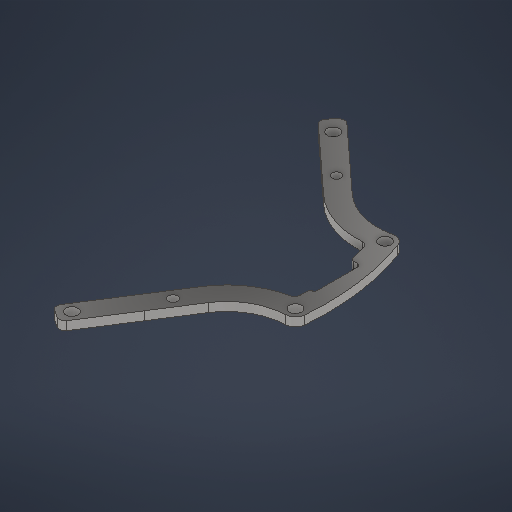
# Autodesk Inventor part: Schwungstrebe
Saved by Autodesk Inventor 2025.2 (Build 292293000, 293)
## iProperties
Created: 2024-05-17
Part Number: Schwungstrebe
Material: Generisch
Document SubType Name: Modeling
Designer: Fabian
Density: 1 g/cm^3
Appearance: Stahl - poliert
Author: Fabian
Autodesk Inventor part; units mm, degrees
ref_plane "YZ Plane" through (0, 0, 0) normal (1, 0, 0) x (0, 1, 0)
ref_plane "XZ Plane" through (0, 0, 0) normal (0, 1, 0) x (-1, 0, 0)
ref_plane "XY Plane" through (0, 0, 0) normal (0, 0, 1) x (1, 0, 0)
sketch "Skizze1" plane through (0, 0, 0) normal (0, 1, 0) x (-1, 0, 0)
  circle A0 centre (-82.6842, 7.2339) radius 2.1
  circle A1 centre (-82.6842, 7.2339) radius 2.1
  circle A2 centre (-77.9945, -28.3877) radius 2.1
  circle A3 centre (-77.9945, -28.3877) radius 2.1
  circle A4 centre (-49.9686, -39.6617) radius 1.6
  circle A5 centre (-49.9686, -39.6617) radius 1.6
  circle A6 centre (-58.5312, 25.3775) radius 1.6
  circle A7 centre (-58.5312, 25.3775) radius 1.6
  line L0 (-51.2809, 30.2441) -> (-59.8777, 16.7498)
  line L1 (-59.8777, 16.7498) -> (-65.7814, 20.5109)
  line L2 (-65.7814, 20.5109) -> (-57.1846, 34.0052)
  line L3 (-57.1846, 34.0052) -> (-51.2809, 30.2441)
  line L4 (-51.2809, 30.2441) -> (-65.7814, 20.5109) construction
  line L5 (-59.8777, 16.7498) -> (-57.1846, 34.0052) construction
  line L6 (13, 63) -> (-13, 63) construction
  line L7 (0, 63) -> (0, -88) construction
  arc A8 (-35.0888, -80.7018) -> (35.0888, -80.7018) centre (0, 0) ccw construction
  line L8 (0, 0) -> (-88, 0) construction
  arc A9 (-85.5688, 20.542) -> (-77.3365, -41.9889) centre (0, 0) ccw construction
  circle A10 centre (-82.6842, 7.2339) radius 3.5
  circle A11 centre (-77.9945, -28.3877) radius 3.5
  line L9 (-41.7058, -42.486) -> (-53.5023, -31.6766)
  line L10 (-53.5023, -31.6766) -> (-58.2314, -36.8375)
  line L11 (-58.2314, -36.8375) -> (-46.4349, -47.6469)
  line L12 (-46.4349, -47.6469) -> (-41.7058, -42.486)
  line L13 (-41.7058, -42.486) -> (-58.2314, -36.8375) construction
  line L14 (-53.5023, -31.6766) -> (-46.4349, -47.6469) construction
  arc A12 (-78.693, 11.2987) -> (-73.0957, -31.2612) centre (0, 0) ccw
  arc A13 (-86.1708, 7.539) -> (-81.2834, -29.5847) centre (0, 0) ccw
  arc A14 (-53.5023, -31.6766) -> (-77.9945, -24.8877) centre (-72.4082, -52.3088) ccw
  arc A15 (-58.2314, -36.8375) -> (-76.7973, -31.6766) centre (-72.5864, -52.5033) ccw
  arc A16 (-82.6842, 3.7339) -> (-59.8777, 16.7498) centre (-83.6316, 31.8827) ccw
  arc A17 (-82.6842, 10.7339) -> (-65.7814, 20.5109) centre (-83.642, 31.8893) ccw
  circle A18 centre (82.6842, 7.2339) radius 2.1
  circle A19 centre (82.6842, 7.2339) radius 2.1
  circle A20 centre (77.9945, -28.3877) radius 2.1
  circle A21 centre (77.9945, -28.3877) radius 2.1
  circle A22 centre (49.9686, -39.6617) radius 1.6
  circle A23 centre (49.9686, -39.6617) radius 1.6
  circle A24 centre (58.5312, 25.3775) radius 1.6
  circle A25 centre (58.5312, 25.3775) radius 1.6
  line L15 (51.2809, 30.2441) -> (59.8777, 16.7498)
  line L16 (59.8777, 16.7498) -> (65.7814, 20.5109)
  line L17 (65.7814, 20.5109) -> (57.1846, 34.0052)
  line L18 (57.1846, 34.0052) -> (51.2809, 30.2441)
  line L19 (51.2809, 30.2441) -> (65.7814, 20.5109) construction
  line L20 (59.8777, 16.7498) -> (57.1846, 34.0052) construction
  arc A26 (77.3365, -41.9889) -> (85.5688, 20.542) centre (0, 0) ccw construction
  circle A27 centre (82.6842, 7.2339) radius 3.5
  circle A28 centre (77.9945, -28.3877) radius 3.5
  line L21 (41.7058, -42.486) -> (53.5023, -31.6766)
  line L22 (53.5023, -31.6766) -> (58.2314, -36.8375)
  line L23 (58.2314, -36.8375) -> (46.4349, -47.6469)
  line L24 (46.4349, -47.6469) -> (41.7058, -42.486)
  line L25 (41.7058, -42.486) -> (58.2314, -36.8375) construction
  line L26 (53.5023, -31.6766) -> (46.4349, -47.6469) construction
  arc A29 (73.0957, -31.2612) -> (78.693, 11.2987) centre (0, 0) ccw
  arc A30 (81.2834, -29.5847) -> (86.1708, 7.539) centre (0, 0) ccw
  arc A31 (77.9945, -24.8877) -> (53.5023, -31.6766) centre (72.4082, -52.3088) ccw
  arc A32 (76.7973, -31.6766) -> (58.2314, -36.8375) centre (72.5864, -52.5033) ccw
  arc A33 (59.8777, 16.7498) -> (82.6842, 3.7339) centre (83.6316, 31.8827) ccw
  arc A34 (65.7814, 20.5109) -> (82.6842, 10.7339) centre (83.642, 31.8893) ccw
  arc A35 (54.3266, 20.6239) -> (52.9459, 20.93) centre (53.4832, 20.0866) ccw
  line L27 (52.9459, 20.93) -> (47.8855, 17.7062)
  arc A36 (47.8855, 17.7062) -> (47.5794, 16.3256) centre (48.4228, 16.8628) ccw
  line L28 (47.5794, 16.3256) -> (56.982, 1.5661)
  arc A37 (56.982, 1.5661) -> (58.3627, 1.26) centre (57.8254, 2.1034) ccw
  line L29 (58.3627, 1.26) -> (63.4231, 4.4838)
  arc A38 (63.4231, 4.4838) -> (63.7292, 5.8644) centre (62.8858, 5.3271) ccw
  line L30 (63.7292, 5.8644) -> (54.3266, 20.6239)
  arc A39 (45.7241, -33.9204) -> (47.137, -33.9821) centre (46.4614, -33.2448) ccw
  line L31 (47.137, -33.9821) -> (60.0395, -22.1594)
  arc A40 (60.0395, -22.1594) -> (60.1012, -20.7466) centre (59.3639, -21.4221) ccw
  line L32 (60.1012, -20.7466) -> (56.0477, -16.3229)
  arc A41 (56.0477, -16.3229) -> (54.6348, -16.2612) centre (55.3104, -16.9984) ccw
  line L33 (54.6348, -16.2612) -> (41.7323, -28.0839)
  arc A42 (41.7323, -28.0839) -> (41.6706, -29.4967) centre (42.4079, -28.8211) ccw
  line L34 (41.6706, -29.4967) -> (45.7241, -33.9204)
  circle A43 centre (30.623, 39.877) radius 2.1
  circle A44 centre (30.1839, -17.0814) radius 2.1
  circle A45 centre (46, -19.5) radius 1.375
  circle A46 centre (40, -19.5) radius 1.375
  circle A47 centre (40, 38.5) radius 1.375
  circle A48 centre (46, 38.5) radius 1.375
  arc A49 (-52.9459, 20.93) -> (-54.3266, 20.6239) centre (-53.4832, 20.0866) ccw
  line L35 (-54.3266, 20.6239) -> (-63.7292, 5.8644)
  arc A50 (-63.7292, 5.8644) -> (-63.4231, 4.4838) centre (-62.8858, 5.3271) ccw
  line L36 (-63.4231, 4.4838) -> (-58.3627, 1.26)
  arc A51 (-58.3627, 1.26) -> (-56.982, 1.5661) centre (-57.8254, 2.1034) ccw
  line L37 (-56.982, 1.5661) -> (-47.5794, 16.3256)
  arc A52 (-47.5794, 16.3256) -> (-47.8855, 17.7062) centre (-48.4228, 16.8628) ccw
  line L38 (-47.8855, 17.7062) -> (-52.9459, 20.93)
  arc A53 (-47.137, -33.9821) -> (-45.7241, -33.9204) centre (-46.4614, -33.2448) ccw
  line L39 (-45.7241, -33.9204) -> (-41.6706, -29.4967)
  arc A54 (-41.6706, -29.4967) -> (-41.7323, -28.0839) centre (-42.4079, -28.8211) ccw
  line L40 (-41.7323, -28.0839) -> (-54.6348, -16.2612)
  arc A55 (-54.6348, -16.2612) -> (-56.0477, -16.3229) centre (-55.3104, -16.9984) ccw
  line L41 (-56.0477, -16.3229) -> (-60.1012, -20.7466)
  arc A56 (-60.1012, -20.7466) -> (-60.0395, -22.1594) centre (-59.3639, -21.4221) ccw
  line L42 (-60.0395, -22.1594) -> (-47.137, -33.9821)
  arc A57 (-74.1912, 7.3101) -> (-74.5045, 6.2355) centre (-72.5045, 6.2355) ccw
  line L43 (-74.1912, 7.3101) -> (-66.8685, 18.8045)
  arc A58 (-66.8685, 18.8045) -> (-66.8312, 18.8624) centre (-71.8916, 22.0861) ccw
  line L44 (-66.8312, 18.8624) -> (-63.3633, 24.3059)
  arc A59 (-63.3633, 24.3059) -> (-63.3633, 24.306) centre (-65.0501, 25.3805) ccw
  line L45 (-63.3633, 24.306) -> (-61.5013, 27.2291)
  arc A60 (-61.5013, 27.2291) -> (-61.5073, 27.2194) centre (-58.5312, 25.3775) ccw
  line L46 (-61.5073, 27.2194) -> (-61.4583, 27.2963)
  arc A61 (-61.4583, 27.2963) -> (-61.4647, 27.2865) centre (-58.5312, 25.3775) ccw
  line L47 (-61.4647, 27.2865) -> (-59.6025, 30.2099)
  arc A62 (-59.6025, 30.2099) -> (-59.5849, 30.2371) centre (-61.2717, 31.3117) ccw
  line L48 (-59.5849, 30.2371) -> (-52.3622, 41.5746)
  arc A63 (-50.6754, 42.5) -> (-52.3622, 41.5746) centre (-50.6754, 40.5) ccw
  line L49 (-50.6754, 42.5) -> (-34.4476, 42.5)
  arc A64 (-34.4476, 42.5) -> (-33.1728, 42.959) centre (-34.4476, 44.5) ccw
  arc A65 (-28.0733, 42.959) -> (-33.1728, 42.959) centre (-30.623, 39.877) ccw
  arc A66 (-28.0733, 42.959) -> (-26.7984, 42.5) centre (-26.7984, 44.5) ccw
  line L50 (-26.7984, 42.5) -> (26.7984, 42.5)
  arc A67 (26.7984, 42.5) -> (28.0733, 42.959) centre (26.7984, 44.5) ccw
  arc A68 (33.1728, 42.959) -> (28.0733, 42.959) centre (30.623, 39.877) ccw
  arc A69 (33.1728, 42.959) -> (34.4476, 42.5) centre (34.4476, 44.5) ccw
  line L51 (34.4476, 42.5) -> (50.6754, 42.5)
  arc A70 (52.3622, 41.5746) -> (50.6754, 42.5) centre (50.6754, 40.5) ccw
  line L52 (52.3622, 41.5746) -> (59.5849, 30.2371)
  arc A71 (59.5849, 30.2371) -> (59.6025, 30.2099) centre (61.2717, 31.3117) ccw
  line L53 (59.6025, 30.2099) -> (61.4647, 27.2865)
  arc A72 (61.4647, 27.2865) -> (61.4583, 27.2963) centre (58.5312, 25.3775) ccw
  line L54 (61.4583, 27.2963) -> (61.5073, 27.2194)
  arc A73 (61.5073, 27.2194) -> (61.5013, 27.2291) centre (58.5312, 25.3775) ccw
  line L55 (61.5013, 27.2291) -> (63.3633, 24.306)
  arc A74 (63.3633, 24.306) -> (63.3633, 24.3059) centre (65.0501, 25.3805) ccw
  line L56 (63.3633, 24.3059) -> (66.8312, 18.8624)
  arc A75 (66.8312, 18.8624) -> (66.8685, 18.8045) centre (71.8916, 22.0861) ccw
  arc A76 (72.5045, -0.25) -> (74.5045, 1.75) centre (72.5045, 1.75) ccw
  line L57 (72.5045, -0.25) -> (63.2545, -0.25)
  arc A77 (63.2545, -0.25) -> (61.2545, -2.25) centre (63.2545, -2.25) ccw
  line L58 (61.2545, -2.25) -> (61.2545, -15.75)
  arc A78 (61.2545, -15.75) -> (63.2545, -17.75) centre (63.2545, -15.75) ccw
  line L59 (63.2545, -17.75) -> (72.5045, -17.75)
  arc A79 (74.5045, -19.75) -> (72.5045, -17.75) centre (72.5045, -19.75) ccw
  line L60 (74.5045, -19.75) -> (74.5045, -21.0459)
  arc A80 (73.8556, -22.5205) -> (74.5045, -21.0459) centre (72.5045, -21.0459) ccw
  arc A81 (51.2741, -42.5) -> (52.6253, -41.9746) centre (51.2741, -40.5) ccw
  line L61 (51.2741, -42.5) -> (-51.2741, -42.5)
  arc A82 (-52.6253, -41.9746) -> (-51.2741, -42.5) centre (-51.2741, -40.5) ccw
  line L62 (-52.6253, -41.9746) -> (-71.5045, -24.675)
  line L63 (-71.5045, -24.675) -> (-73.8556, -22.5205)
  arc A83 (-74.5045, -21.0459) -> (-73.8556, -22.5205) centre (-72.5045, -21.0459) ccw
  line L64 (-74.5045, -21.0459) -> (-74.5045, -19.75)
  arc A84 (-72.5045, -17.75) -> (-74.5045, -19.75) centre (-72.5045, -19.75) ccw
  line L65 (-72.5045, -17.75) -> (-63.2545, -17.75)
  arc A85 (-63.2545, -17.75) -> (-61.2545, -15.75) centre (-63.2545, -15.75) ccw
  line L66 (-61.2545, -15.75) -> (-61.2545, -2.25)
  arc A86 (-61.2545, -2.25) -> (-63.2545, -0.25) centre (-63.2545, -2.25) ccw
  line L67 (-63.2545, -0.25) -> (-72.5045, -0.25)
  arc A87 (-74.5045, 1.75) -> (-72.5045, -0.25) centre (-72.5045, 1.75) ccw
  line L68 (-74.5045, 1.75) -> (-74.5045, 6.2355)
  circle A88 centre (-46, 38.5) radius 1.375
  circle A89 centre (-40, 38.5) radius 1.375
  circle A90 centre (-40, -19.5) radius 1.375
  circle A91 centre (-46, -19.5) radius 1.375
  circle A92 centre (-30.1839, -17.0814) radius 2.1
  circle A93 centre (-30.623, 39.877) radius 2.1
  line L69 (44.0704, -45.0665) -> (38.9094, -49.7956) construction
  line L70 (47.6229, 42.5) -> (43.8618, 48.4037) construction
  line L71 (-47.6229, 42.5) -> (-43.8618, 48.4037) construction
  line L72 (-44.0704, -45.0665) -> (-38.9094, -49.7956) construction
  line L73 (31.3839, -51.9443) -> (41.7058, -42.486)
  line L74 (41.7058, -42.486) -> (46.4349, -47.6469)
  line L75 (46.4349, -47.6469) -> (36.1131, -57.1052)
  line L76 (36.1131, -57.1052) -> (31.3839, -51.9443)
  line L77 (31.3839, -51.9443) -> (46.4349, -47.6469) construction
  line L78 (41.7058, -42.486) -> (36.1131, -57.1052) construction
  line L79 (-31.3839, -51.9442) -> (-41.7058, -42.486)
  line L80 (-41.7058, -42.486) -> (-46.435, -47.647)
  line L81 (-46.435, -47.647) -> (-36.1131, -57.1052)
  line L82 (-36.1131, -57.1052) -> (-31.3839, -51.9442)
  line L83 (-31.3839, -51.9442) -> (-46.435, -47.647) construction
  line L84 (-41.7058, -42.486) -> (-36.1131, -57.1052) construction
  line L85 (38.9094, -49.7956) -> (33.7485, -54.5247)
  circle A94 centre (36.329, -52.1602) radius 2
  line L86 (33.7485, -54.5247) -> (32.2739, -55.8759)
  line L87 (32.2739, -55.8759) -> (34.6385, -58.4564)
  line L88 (34.6385, -58.4564) -> (36.1131, -57.1052)
  line L89 (32.2739, -55.8759) -> (29.9094, -53.2954)
  line L90 (29.9094, -53.2954) -> (31.3839, -51.9443)
  line L91 (-36.1131, -57.1052) -> (-31.3839, -51.9443)
  circle A95 centre (-36.329, -52.1602) radius 2
  line L92 (-33.7485, -54.5247) -> (-32.2739, -55.8759)
  line L93 (-32.2739, -55.8759) -> (-34.6385, -58.4564)
  line L94 (-34.6385, -58.4564) -> (-36.1131, -57.1052)
  line L95 (-32.2739, -55.8759) -> (-29.9094, -53.2954)
  line L96 (-29.9094, -53.2954) -> (-31.3839, -51.9443)
  line L97 (-40.9067, 53.0424) -> (-37.9548, 51.1618)
  line L98 (-37.9548, 51.1618) -> (-51.2809, 30.2441)
  line L99 (-40.9067, 53.0424) -> (-43.8585, 54.9229)
  line L100 (-43.8585, 54.9229) -> (-57.1846, 34.0052)
  circle A96 centre (-44.9364, 46.717) radius 2
  line L101 (-44.9364, 46.717) -> (-42.7872, 50.0905)
  line L102 (-42.7872, 50.0905) -> (-39.8354, 48.21)
  line L103 (-42.7872, 50.0905) -> (-45.7391, 51.9711)
  circle A97 centre (-44.9364, 46.717) radius 2.1
  circle A98 centre (-36.329, -52.1602) radius 2.1
  point P0 (0, 0)
  point P1 (-75.6274, -24.5102)
  point P2 (-79.3974, 4.0381)
  point P3 (-86.1708, 7.539)
  point P4 (-81.2834, -29.5847)
  point P5 (88, 0)
  point P6 (-41.6905, -42.5)
  point P7 (-41.7186, -42.5)
  dimension "d0" = 16
  dimension "d1" = 7
  dimension "d2" = 7
  dimension "d3" = 16
  dimension "d4" = 7
  dimension "d42" = 7
  dimension "d43" = 7
  dimension "d46" = 4
  dimension "d47" = 2
  dimension "d50" = 3.5
  dimension "d51" = 3.5
  dimension "d53" = 4
  dimension "d54" = 4
  dimension "d55" = 4.2
  dimension "d56" = 4.2
  constraints: 208 end point, 143 point on circle, 99 centre point, 40 symmetric about line, 22 coincident, 15 midpoint, 9 parallel, 9 perpendicular, 7 point on line, 5 tangent, 1 horizontal, 1 vertical, 18 other
  measures "d0" distance of L0.start L0.end
  measures "d1" diameter of A10
  measures "d2" diameter of A11
  measures "d3" distance of L9.start L9.end
  measures "d4" radial gap between concentric circles of A13 A12
  measures "d42" distance of L69.start L69.end
  measures "d43" distance of L70.start L70.end
  measures "d46" diameter of A94
  measures "d47" distance of L85.end L86.end
  measures "d50" distance of L97.start L97.end
  measures "d51" distance of L97.start L99.end
  measures "d53" diameter of A96
  measures "d54" distance of L101.start L101.end
  measures "d55" diameter of A97
  measures "d56" diameter of A98
extrude "Extrusion1" add sketch "Skizze1" along normal blind 3 contours L0 L1 L2 L3 | L3 L48 A63 L49 L98 A88 | A16 L68 A57 L43 A58 L44 L1 | A88 L98 | L44 A58 L43 A57 L68 A16 A12 A17 | L100 L103 L102 L98 L49 A63 | A12 A10 A17 | A16 A10 A12 | A12 A14 A11 A13 A10 A16 | A10 | A14 L63 L62 A15 A12 | A12 A11 A14 | A12 A15 A11 | A11 | A14 L10 L62 L63 | L9 L12 L61 A82 L11 L10 | L79 L61 L12 | A82 L61 L12 L11 | L61 L79 L82 L81 L12 | L96 L95 L92 L82 | L82 L92 L93 L94 picked at (-46.5547, 39.0575)
fillet "Rundung1" radius 2 6 edges at (79.3974, 1.5, 4.0381) (75.6274, 1.5, -24.5102) (29.9094, 1.5, -53.2954) (34.6385, 1.5, -58.4564) (45.7391, 1.5, 51.9711) (39.8354, 1.5, 48.21)
sketch "Skizze2" plane through (0, 3, 0) normal (0, 1, 0) x (1, 0, 0)
  line L0 (19.0016, 59.2215) -> (57.3401, 24.0908)
  arc A0 (57.3401, 24.0908) -> (69.3003, 22.9246) centre (64.096, 31.4636) ccw
  arc A1 (75.2406, 20.5635) -> (69.3003, 22.9246) centre (71.3821, 19.509) ccw
  arc A2 (77.999, -0.3892) -> (75.2406, 20.5635) centre (0, 0) ccw
  arc A3 (72.8723, -4.2072) -> (77.999, -0.3892) centre (73.9991, -0.3692) ccw
  arc A4 (72.8723, -4.2072) -> (61.6214, -8.4293) centre (70.0553, -13.8022) ccw
  line L1 (61.6214, -8.4293) -> (37.5911, -46.1492)
  arc A5 (34.2176, -48) -> (37.5911, -46.1492) centre (34.2176, -44) ccw
  line L2 (34.2176, -48) -> (29, -48)
  arc A6 (29, -48) -> (25.0078, -51.75) centre (29, -52) ccw
  arc A7 (21.0156, -55.5) -> (25.0078, -51.75) centre (21.0156, -51.5) ccw
  line L3 (21.0156, -55.5) -> (-21.0156, -55.5)
  circle A8 centre (36.75, -68) radius 1.8
  circle A9 centre (36.75, -61) radius 1.8
  circle A10 centre (36.75, -54) radius 1.8
  line L4 (30.1812, 62.5407) -> (59.6723, 35.5171)
  arc A11 (59.6723, 35.5171) -> (68.1495, 35.8873) centre (63.7258, 39.9408) ccw
  line L5 (68.1495, 35.8873) -> (74.1043, 42.3858)
  arc A12 (77.3365, 41.9889) -> (74.1043, 42.3858) centre (75.5788, 41.0346) ccw
  arc A13 (85.5688, -20.542) -> (77.3365, 41.9889) centre (0, 0) ccw
  arc A14 (82.5495, -21.7619) -> (85.5688, -20.542) centre (83.6241, -20.0751) ccw
  line L6 (82.5495, -21.7619) -> (75.1157, -17.026)
  arc A15 (75.1157, -17.026) -> (66.8315, -18.8626) centre (71.8919, -22.0864) ccw
  line L7 (66.8315, -18.8626) -> (45.3395, -52.5983)
  arc A16 (45.3395, -52.5983) -> (47.1761, -60.8824) centre (50.3999, -55.8221) ccw
  line L8 (47.1761, -60.8824) -> (54.6099, -65.6183)
  arc A17 (54.7803, -68.8703) -> (54.6099, -65.6183) centre (53.5353, -67.3051) ccw
  arc A18 (44.8368, -75.7209) -> (54.7803, -68.8703) centre (0, 0) ccw
  arc A19 (43.8178, -76) -> (44.8368, -75.7209) centre (43.8178, -74) ccw
  line L9 (43.8178, -76) -> (35.75, -76)
  arc A20 (33.75, -74) -> (35.75, -76) centre (35.75, -74) ccw
  line L10 (33.75, -74) -> (33.75, -64)
  arc A21 (33.75, -64) -> (30.0179, -63) centre (31.75, -64) ccw
  arc A22 (28.2859, -64) -> (30.0179, -63) centre (28.2859, -62) ccw
  line L11 (28.2859, -64) -> (14.7321, -64)
  circle A23 centre (49.9686, 39.6617) radius 1.8
  circle A24 centre (55.4982, 34.5948) radius 1.8
  circle A25 centre (58.5312, -25.3775) radius 1.8
  circle A26 centre (54.5014, -31.7029) radius 1.8
  circle A27 centre (62.5609, -19.052) radius 1.8
  line L12 (37.1695, -45.8805) -> (61.1997, -8.1606)
  arc A28 (73.0131, -3.7275) -> (61.1997, -8.1606) centre (70.0553, -13.8022) ccw
  arc A29 (73.0131, -3.7275) -> (77.499, -0.3867) centre (73.9991, -0.3692) ccw
  arc A30 (77.499, -0.3867) -> (74.7582, 20.4317) centre (0, 0) ccw
  arc A31 (74.7582, 20.4317) -> (69.5605, 22.4976) centre (71.3821, 19.509) ccw
  arc A32 (57.0023, 23.7222) -> (69.5605, 22.4976) centre (64.096, 31.4636) ccw
  line L13 (57.0023, 23.7222) -> (18.6638, 58.8529)
  line L14 (-21.0156, -55) -> (21.0156, -55)
  arc A33 (21.0156, -55) -> (24.5088, -51.7188) centre (21.0156, -51.5) ccw
  arc A34 (29, -47.5) -> (24.5088, -51.7188) centre (29, -52) ccw
  line L15 (29, -47.5) -> (34.2176, -47.5)
  arc A35 (34.2176, -47.5) -> (37.1695, -45.8805) centre (34.2176, -44) ccw
  line L16 (47.604, 37.0813) -> (31.5682, 51.7754)
  line L17 (31.5682, 51.7754) -> (63.6398, 22.3872)
  line L18 (63.6398, 22.3872) -> (50.128, 7.6416)
  line L19 (47.3023, 7.5183) -> (18.1798, 34.2041)
  line L20 (18.0564, 37.0298) -> (31.5682, 51.7754)
  line L21 (58.5312, -25.3775) -> (55.5793, -23.4969)
  line L22 (55.5793, -23.4969) -> (67.2656, -5.1532)
  line L23 (67.2656, -5.1532) -> (43.893, -41.8407)
  line L24 (43.893, -41.8407) -> (27.0252, -31.0947)
  line L25 (26.413, -28.3333) -> (47.6364, 4.9806)
  line L26 (50.3977, 5.5928) -> (67.2656, -5.1532)
  arc A36 (50.3977, 5.5928) -> (47.6364, 4.9806) centre (49.3231, 3.906) ccw
  arc A37 (47.3023, 7.5183) -> (50.128, 7.6416) centre (48.6535, 8.9928) ccw
  arc A38 (26.413, -28.3333) -> (27.0252, -31.0947) centre (28.0998, -29.4079) ccw
  line L27 (81.0045, 17) -> (62.0045, 17)
  line L28 (62.0045, 17) -> (62.0045, 1)
  line L29 (62.0045, 1) -> (81.0045, 1)
  line L30 (81.0045, 1) -> (81.0045, 17)
  line L31 (81.0045, 17) -> (62.0045, 1) construction
  line L32 (62.0045, 17) -> (81.0045, 1) construction
  arc A39 (-37.5911, -46.1492) -> (-34.2176, -48) centre (-34.2176, -44) ccw
  line L33 (-37.5911, -46.1492) -> (-61.6214, -8.4293)
  arc A40 (-61.6214, -8.4293) -> (-72.8723, -4.2072) centre (-70.0553, -13.8022) ccw
  arc A41 (-77.999, -0.3892) -> (-72.8723, -4.2072) centre (-73.9991, -0.3692) ccw
  arc A42 (-75.2406, 20.5635) -> (-77.999, -0.3892) centre (0, 0) ccw
  arc A43 (-69.3003, 22.9246) -> (-75.2406, 20.5635) centre (-71.3821, 19.509) ccw
  arc A44 (-69.3003, 22.9246) -> (-57.3401, 24.0908) centre (-64.096, 31.4636) ccw
  line L34 (-57.3401, 24.0908) -> (-19.0016, 59.2215)
  arc A45 (-19.0016, 59.2215) -> (-16.7974, 71.0346) centre (-25.7575, 66.5943) ccw
  arc A46 (-13.9276, 76.7465) -> (-16.7974, 71.0346) centre (-13.2134, 72.8108) ccw
  arc A47 (13.9276, 76.7465) -> (-13.9276, 76.7465) centre (0, 0) ccw
  arc A48 (16.7974, 71.0346) -> (13.9276, 76.7465) centre (13.2134, 72.8108) ccw
  arc A49 (16.7974, 71.0346) -> (19.0016, 59.2215) centre (25.7575, 66.5943) ccw
  line L35 (19.0016, 59.2215) -> (57.3401, 24.0908)
  arc A50 (57.3401, 24.0908) -> (69.3003, 22.9246) centre (64.096, 31.4636) ccw
  arc A51 (75.2406, 20.5635) -> (69.3003, 22.9246) centre (71.3821, 19.509) ccw
  arc A52 (77.999, -0.3892) -> (75.2406, 20.5635) centre (0, 0) ccw
  arc A53 (72.8723, -4.2072) -> (77.999, -0.3892) centre (73.9991, -0.3692) ccw
  arc A54 (72.8723, -4.2072) -> (61.6214, -8.4293) centre (70.0553, -13.8022) ccw
  line L36 (61.6214, -8.4293) -> (37.5911, -46.1492)
  arc A55 (34.2176, -48) -> (37.5911, -46.1492) centre (34.2176, -44) ccw
  line L37 (34.2176, -48) -> (29, -48)
  arc A56 (29, -48) -> (25.0078, -51.75) centre (29, -52) ccw
  arc A57 (21.0156, -55.5) -> (25.0078, -51.75) centre (21.0156, -51.5) ccw
  line L38 (21.0156, -55.5) -> (-21.0156, -55.5)
  arc A58 (-25.0078, -51.75) -> (-21.0156, -55.5) centre (-21.0156, -51.5) ccw
  arc A59 (-25.0078, -51.75) -> (-29, -48) centre (-29, -52) ccw
  line L39 (-29, -48) -> (-34.2176, -48)
  circle A60 centre (-24.9586, 79.1585) radius 2.8
  circle A61 centre (-76.682, 31.7627) radius 2.8
  circle A62 centre (-82.2899, -10.8337) radius 2.8
  circle A63 centre (-36.75, -68) radius 1.8
  circle A64 centre (-36.75, -61) radius 1.8
  circle A65 centre (-36.75, -54) radius 1.8
  circle A66 centre (-49.9686, 39.6617) radius 1.8
  circle A67 centre (-55.4982, 34.5948) radius 1.8
  circle A68 centre (-44.439, 44.7287) radius 1.8
  circle A69 centre (-62.5609, -19.052) radius 1.8
  circle A70 centre (-54.5014, -31.7029) radius 1.8
  circle A71 centre (-58.5312, -25.3775) radius 1.8
  circle A72 centre (36.75, -68) radius 1.8
  circle A73 centre (36.75, -61) radius 1.8
  circle A74 centre (36.75, -54) radius 1.8
  circle A75 centre (24.9586, 79.1585) radius 2.8
  arc A76 (29.8111, 71.018) -> (30.1812, 62.5407) centre (34.2347, 66.9644) ccw
  line L40 (30.1812, 62.5407) -> (59.6723, 35.5171)
  arc A77 (59.6723, 35.5171) -> (68.1495, 35.8873) centre (63.7258, 39.9408) ccw
  line L41 (68.1495, 35.8873) -> (74.1043, 42.3858)
  arc A78 (77.3365, 41.9889) -> (74.1043, 42.3858) centre (75.5788, 41.0346) ccw
  arc A79 (85.5688, -20.542) -> (77.3365, 41.9889) centre (0, 0) ccw
  arc A80 (82.5495, -21.7619) -> (85.5688, -20.542) centre (83.6241, -20.0751) ccw
  line L42 (82.5495, -21.7619) -> (75.1157, -17.026)
  arc A81 (75.1157, -17.026) -> (66.8315, -18.8626) centre (71.8919, -22.0864) ccw
  line L43 (66.8315, -18.8626) -> (45.3395, -52.5983)
  arc A82 (45.3395, -52.5983) -> (47.1761, -60.8824) centre (50.3999, -55.8221) ccw
  line L44 (47.1761, -60.8824) -> (54.6099, -65.6183)
  arc A83 (54.7803, -68.8703) -> (54.6099, -65.6183) centre (53.5353, -67.3051) ccw
  arc A84 (44.8368, -75.7209) -> (54.7803, -68.8703) centre (0, 0) ccw
  arc A85 (43.8178, -76) -> (44.8368, -75.7209) centre (43.8178, -74) ccw
  line L45 (43.8178, -76) -> (35.75, -76)
  arc A86 (33.75, -74) -> (35.75, -76) centre (35.75, -74) ccw
  line L46 (33.75, -74) -> (33.75, -64)
  arc A87 (33.75, -64) -> (30.0179, -63) centre (31.75, -64) ccw
  arc A88 (28.2859, -64) -> (30.0179, -63) centre (28.2859, -62) ccw
  line L47 (28.2859, -64) -> (14.7321, -64)
  arc A89 (13, -63) -> (14.7321, -64) centre (14.7321, -62) ccw
  line L48 (-14.7321, -64) -> (-28.2859, -64)
  arc A90 (-30.0179, -63) -> (-28.2859, -64) centre (-28.2859, -62) ccw
  arc A91 (-30.0179, -63) -> (-33.75, -64) centre (-31.75, -64) ccw
  line L49 (-33.75, -64) -> (-33.75, -74)
  arc A92 (-35.75, -76) -> (-33.75, -74) centre (-35.75, -74) ccw
  line L50 (-35.75, -76) -> (-43.8178, -76)
  arc A93 (-44.8368, -75.7209) -> (-43.8178, -76) centre (-43.8178, -74) ccw
  arc A94 (-54.7803, -68.8703) -> (-44.8368, -75.7209) centre (0, 0) ccw
  arc A95 (-54.6099, -65.6183) -> (-54.7803, -68.8703) centre (-53.5353, -67.3051) ccw
  line L51 (-54.6099, -65.6183) -> (-47.1761, -60.8824)
  arc A96 (-47.1761, -60.8824) -> (-45.3395, -52.5983) centre (-50.3999, -55.8221) ccw
  line L52 (-45.3395, -52.5983) -> (-66.8315, -18.8626)
  arc A97 (-66.8315, -18.8626) -> (-75.1157, -17.026) centre (-71.8919, -22.0864) ccw
  line L53 (-75.1157, -17.026) -> (-82.5495, -21.7619)
  arc A98 (-85.5688, -20.542) -> (-82.5495, -21.7619) centre (-83.6241, -20.0751) ccw
  arc A99 (-77.3365, 41.9889) -> (-85.5688, -20.542) centre (0, 0) ccw
  arc A100 (-74.1043, 42.3858) -> (-77.3365, 41.9889) centre (-75.5788, 41.0346) ccw
  line L54 (-74.1043, 42.3858) -> (-68.1495, 35.8873)
  arc A101 (-68.1495, 35.8873) -> (-59.6723, 35.5171) centre (-63.7258, 39.9408) ccw
  line L55 (-59.6723, 35.5171) -> (-30.1812, 62.5407)
  arc A102 (-30.1812, 62.5407) -> (-29.8111, 71.018) centre (-34.2347, 66.9644) ccw
  line L56 (-29.8111, 71.018) -> (-35.7659, 77.5165)
  arc A103 (-35.0888, 80.7018) -> (-35.7659, 77.5165) centre (-34.2913, 78.8676) ccw
  arc A104 (35.0888, 80.7018) -> (-35.0888, 80.7018) centre (0, 0) ccw
  arc A105 (35.7659, 77.5165) -> (35.0888, 80.7018) centre (34.2913, 78.8676) ccw
  line L57 (35.7659, 77.5165) -> (29.8111, 71.018)
  circle A106 centre (49.9686, 39.6617) radius 1.8
  circle A107 centre (55.4982, 34.5948) radius 1.8
  circle A108 centre (58.5312, -25.3775) radius 1.8
  circle A109 centre (54.5014, -31.7029) radius 1.8
  circle A110 centre (44.439, 44.7287) radius 1.8
  circle A111 centre (62.5609, -19.052) radius 1.8
  line L58 (37.1695, -45.8805) -> (61.1997, -8.1606)
  arc A112 (73.0131, -3.7275) -> (61.1997, -8.1606) centre (70.0553, -13.8022) ccw
  arc A113 (73.0131, -3.7275) -> (77.499, -0.3867) centre (73.9991, -0.3692) ccw
  arc A114 (77.499, -0.3867) -> (74.7582, 20.4317) centre (0, 0) ccw
  arc A115 (74.7582, 20.4317) -> (69.5605, 22.4976) centre (71.3821, 19.509) ccw
  arc A116 (57.0023, 23.7222) -> (69.5605, 22.4976) centre (64.096, 31.4636) ccw
  line L59 (57.0023, 23.7222) -> (18.6638, 58.8529)
  arc A117 (16.3494, 71.2566) -> (18.6638, 58.8529) centre (25.7575, 66.5943) ccw
  arc A118 (16.3494, 71.2566) -> (13.8384, 76.2545) centre (13.2134, 72.8108) ccw
  arc A119 (13.8384, 76.2545) -> (-13.8384, 76.2545) centre (0, 0) ccw
  arc A120 (-13.8384, 76.2545) -> (-16.3494, 71.2566) centre (-13.2134, 72.8108) ccw
  arc A121 (-18.6638, 58.8529) -> (-16.3494, 71.2566) centre (-25.7575, 66.5943) ccw
  line L60 (-18.6638, 58.8529) -> (-57.0023, 23.7222)
  arc A122 (-69.5605, 22.4976) -> (-57.0023, 23.7222) centre (-64.096, 31.4636) ccw
  arc A123 (-69.5605, 22.4976) -> (-74.7582, 20.4317) centre (-71.3821, 19.509) ccw
  arc A124 (-74.7582, 20.4317) -> (-77.499, -0.3867) centre (0, 0) ccw
  arc A125 (-77.499, -0.3867) -> (-73.0131, -3.7275) centre (-73.9991, -0.3692) ccw
  arc A126 (-61.1997, -8.1606) -> (-73.0131, -3.7275) centre (-70.0553, -13.8022) ccw
  line L61 (-61.1997, -8.1606) -> (-37.1695, -45.8805)
  arc A127 (-37.1695, -45.8805) -> (-34.2176, -47.5) centre (-34.2176, -44) ccw
  line L62 (-34.2176, -47.5) -> (-29, -47.5)
  arc A128 (-24.5088, -51.7188) -> (-29, -47.5) centre (-29, -52) ccw
  arc A129 (-24.5088, -51.7188) -> (-21.0156, -55) centre (-21.0156, -51.5) ccw
  line L63 (-21.0156, -55) -> (21.0156, -55)
  arc A130 (21.0156, -55) -> (24.5088, -51.7188) centre (21.0156, -51.5) ccw
  arc A131 (29, -47.5) -> (24.5088, -51.7188) centre (29, -52) ccw
  line L64 (29, -47.5) -> (34.2176, -47.5)
  arc A132 (34.2176, -47.5) -> (37.1695, -45.8805) centre (34.2176, -44) ccw
  circle A133 centre (16, 9) radius 2.1
  line L65 (-19, -53) -> (-19, 12)
  circle A134 centre (4, 47) radius 1.621
  circle A135 centre (-4, 47) radius 1.621
  arc A136 (7, 49.9161) -> (10.3333, 45.972) centre (11, 49.9161) ccw
  arc A137 (12, 44) -> (10.3333, 45.972) centre (10, 44) ccw
  line L66 (12, 44) -> (12, -5)
  line L67 (12, -5) -> (10, -5)
  arc A138 (8, -3) -> (10, -5) centre (10, -3) ccw
  line L68 (8, -3) -> (8, 1)
  arc A139 (8, 1) -> (6, 3) centre (6, 1) ccw
  line L69 (6, 3) -> (-6, 3)
  arc A140 (-6, 3) -> (-8, 1) centre (-6, 1) ccw
  line L70 (-8, 1) -> (-8, -3)
  arc A141 (-10, -5) -> (-8, -3) centre (-10, -3) ccw
  line L71 (-10, -5) -> (-12, -5)
  line L72 (-12, -5) -> (-12, 44)
  arc A142 (-10.3333, 45.972) -> (-12, 44) centre (-10, 44) ccw
  arc A143 (-10.3333, 45.972) -> (-7, 49.9161) centre (-11, 49.9161) ccw
  line L73 (-7, 49.9161) -> (-7, 54)
  arc A144 (-5, 56) -> (-7, 54) centre (-5, 54) ccw
  line L74 (-5, 56) -> (5, 56)
  arc A145 (7, 54) -> (5, 56) centre (5, 54) ccw
  line L75 (7, 54) -> (7, 49.9161)
  line L76 (-13, -63) -> (13, -63) construction
  line L77 (0, -63) -> (0, 88) construction
  arc A146 (35.0888, 80.7018) -> (-35.0888, 80.7018) centre (0, 0) ccw construction
  line L78 (0, 0) -> (88, 0) construction
  arc A147 (85.5688, -20.542) -> (77.3365, 41.9889) centre (0, 0) ccw construction
  circle A148 centre (0, 0) radius 75 construction
  line L79 (0, 0) -> (70.4769, 25.6515) construction
  line L80 (0, 0) -> (74.7146, -6.5367) construction
  circle A149 centre (0, 0) radius 78
  circle A150 centre (70.4769, 25.6515) radius 3
  circle A151 centre (74.7146, -6.5367) radius 3
  circle A152 centre (0, 0) radius 72
  arc A153 (29, -48) -> (25.0078, -51.75) centre (29, -52) ccw construction
  circle A154 centre (29, -52) radius 3.5
  line L81 (34.2176, -48) -> (29, -48) construction
  line L82 (29, -55.5) -> (21.0156, -55.5)
  circle A155 centre (29, -52) radius 4
  line L83 (32.5, -48) -> (29, -48)
  arc A156 (21.0156, -55.5) -> (25.0078, -51.75) centre (21.0156, -51.5) ccw
  arc A157 (21.0156, -55.5) -> (25.0078, -51.75) centre (21.0156, -51.5) ccw
  line L84 (32.5, -52) -> (32.5, -48)
  circle A158 centre (74.7146, -6.5367) radius 1.6
  circle A159 centre (70.4769, 25.6515) radius 1.6
  circle A160 centre (29, -52) radius 1.6
  line L85 (0, -55.5) -> (0, 88)
  line L86 (84.0045, -2) -> (59.0045, -2)
  line L87 (59.0045, -2) -> (59.0045, 20)
  line L88 (59.0045, 20) -> (84.0045, 20)
  line L89 (84.0045, 20) -> (84.0045, -2)
  line L90 (74.7146, -6.5367) -> (74.7146, 9.8771) construction
  line L91 (78.7146, -6.5367) -> (78.7146, 9.8771)
  line L92 (70.7146, 9.8771) -> (70.7146, -6.5367)
  arc A161 (70.7146, -6.5367) -> (78.7146, -6.5367) centre (74.7146, -6.5367) ccw
  arc A162 (78.7146, 9.8771) -> (70.7146, 9.8771) centre (74.7146, 9.8771) ccw
  line L93 (70.4769, 25.6515) -> (70.4769, 13.0481) construction
  line L94 (66.4769, 25.6515) -> (66.4769, 13.0481)
  line L95 (74.4769, 13.0481) -> (74.4769, 25.6515)
  arc A163 (74.4769, 25.6515) -> (66.4769, 25.6515) centre (70.4769, 25.6515) ccw
  arc A164 (66.4769, 13.0481) -> (74.4769, 13.0481) centre (70.4769, 13.0481) ccw
  point P0 (-138.8202, 84.2178)
  point P1 (0, 0)
  point P2 (-120.3366, -136.1149)
  point P3 (-153.6172, -136.1149)
  point P4 (-152.3366, -136.1149)
  point P5 (-121.6172, -136.1149)
  point P6 (48.7768, 6.1671)
  point P7 (25.3384, -30.0201)
  point P8 (-138.8202, 84.2178)
  point P9 (-138.8202, 84.2178)
  point P10 (20.9734, 5.2463)
  point P11 (-12.3073, 5.2463)
  point P12 (-11.0266, 5.2463)
  point P13 (19.6927, 5.2463)
  point P14 (-138.8202, 79.2178)
  point P15 (0, 56)
  point P16 (159.5559, 30.6223)
  point P17 (153.5787, 31.1452)
  point P18 (157.9859, -2.3305)
  point P19 (163.624, -0.2784)
  point P20 (202.2819, 72.3471)
  point P21 (206.2741, 76.0971)
  point P22 (77.6291, 86.9239)
  point P23 (71.9909, 84.8718)
  point P24 (72.7458, 82.6897)
  point P25 (25.3487, 4.7463)
  point P26 (36.8331, 12.2463)
  point P27 (76.2234, 56.2743)
  point P28 (76.0591, 53.9711)
  point P29 (82.0362, 53.4482)
  point P30 (82.3321, 59.8572)
  point P31 (79.5736, 80.8099)
  point P32 (4.3331, 138.2463)
  point P33 (4.3331, 116.2463)
  point P34 (4.3331, 72.2463)
  point P35 (4.3331, 69.2463)
  point P36 (4.3331, 4.7463)
  point P37 (74.7146, 1.6702)
  point P38 (70.4769, 19.3498)
  point P39 (-265.923, 167.47)
  point P40 (-257.923, 167.47)
  point P41 (-270.1607, 189.47)
  point P42 (-262.1607, 189.47)
  point P43 (76.1249, 17)
  point P44 (76.8665, 13.249)
  point P45 (78.7146, 1)
  dimension "d8" = 0.5
  dimension "d9" = 43.5
  dimension "d10" = 22
  dimension "d11" = 3.5
  dimension "d12" = 21.75
  dimension "d13" = 43.5
  dimension "d14" = 22
  dimension "d15" = 2
  dimension "d16" = 19
  dimension "d17" = 16
  dimension "d18" = 1
  dimension "d19" = 0.5
  dimension "d20" = 4.2
  dimension "d21" = 65
  dimension "d22" = 150
  dimension "d23" = 20
  dimension "d24" = 5
  dimension "d25" = 156
  dimension "d26" = 6
  dimension "d27" = 6
  dimension "d28" = 7
  dimension "d29" = 4
  dimension "d30" = 3.2
  dimension "d31" = 3.2
  dimension "d32" = 3.2
  dimension "d33" = 3
  dimension "d35" = 8
  dimension "d36" = 8
  constraints: 250 point on circle, 196 end point, 165 centre point, 16 tangent, 13 coincident, 11 parallel, 7 perpendicular, 7 point on line, 5 midpoint, 2 collinear, 2 equal radius, 1 concentric, 1 vertical, 40 other
  measures "d8" distance between parallel lines of L1 L12
  measures "d9" distance of L16.end L17.end
  measures "d10" distance of L17.end point (48.777, 6.167)
  measures "d11" distance of L21.start L21.end
  measures "d12" distance of L21.end L22.end
  measures "d13" distance of L22.end L23.end
  measures "d14" distance of L23.end point (25.338, -30.02)
  measures "d15" radius of A36
  measures "d16" distance of L29.end L28.end
  measures "d17" distance of L28.end L27.end
  measures "d18" distance from line of L29 point (0, 0)
  measures "d19" distance between parallel lines of L36 L58
  measures "d20" diameter of A133
  measures "d21" distance of L65.start L65.end
  measures "d22" diameter of A148
  measures "d23" angle of L78 L79
  measures "d24" angle of L78 L80
  measures "d25" diameter of A149
  measures "d26" diameter of A150
  measures "d27" diameter of A151
  measures "d28" diameter of A154
  measures "d29" distance of L84.start L83.start
  measures "d30" diameter of A158
  measures "d31" diameter of A159
  measures "d32" diameter of A160
  measures "d33" distance between parallel lines of L29 L86
  measures "d35" diameter of A162
  measures "d36" diameter of A164
extrude "Extrusion2" cut sketch "Skizze2" against normal blind 3 contours L27 L30 L29 L91 A162 A2
fillet "Rundung2" radius 1 4 edges at (77.6611, 1.5, -17) (79.4937, 1.5, -1) (81.0045, 1.5, -17) (81.0045, 1.5, -1)
